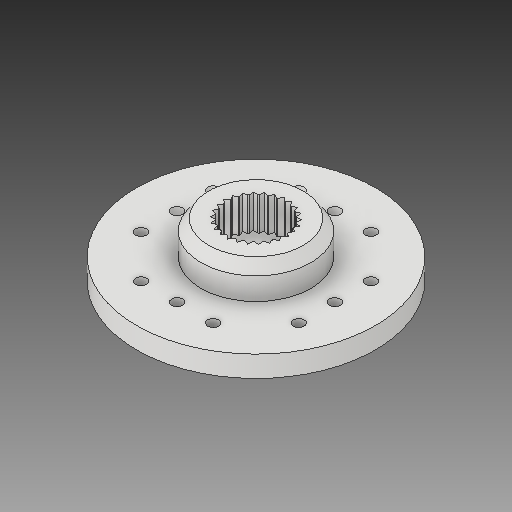
# Autodesk Inventor part: Acople circular
Saved by Autodesk Inventor 2019 (Build 230136000, 136)
## iProperties
Created: 2016-09-27
Part Number: Acople circular
Material: Plástico ABS
Document SubType Name: Modeling
Designer: Julian
Density: 1.06 g/cm^3
Appearance: Suave - Blanco
Mass: 0.859637 g
Surface Area: 11.1715 cm^2
Volume: 0.810978 cm^3
Author: Julian
Autodesk Inventor part; units mm, degrees
ref_plane "YZ Plane" through (0, 0, 0) normal (1, 0, 0) x (0, 1, 0)
ref_plane "XZ Plane" through (0, 0, 0) normal (0, 1, 0) x (-1, 0, 0)
ref_plane "XY Plane" through (0, 0, 0) normal (0, 0, 1) x (1, 0, 0)
sketch "Boceto1" plane through (0, 0, 0) normal (0, 1, 0) x (-1, 0, 0)
  circle A0 centre (0, 0) radius 10.75
  circle A1 centre (7.1, 0) radius 0.5
  circle A2 centre (7.1, -3.25) radius 0.5
  circle A3 centre (7.1, 3.25) radius 0.5
  circle A4 centre (-3.25, 7.1) radius 0.5
  circle A5 centre (0, 7.1) radius 0.5
  circle A6 centre (3.25, 7.1) radius 0.5
  circle A7 centre (-7.1, -3.25) radius 0.5
  circle A8 centre (-7.1, 0) radius 0.5
  circle A9 centre (-7.1, 3.25) radius 0.5
  circle A10 centre (3.25, -7.1) radius 0.5
  circle A11 centre (0, -7.1) radius 0.5
  circle A12 centre (-3.25, -7.1) radius 0.5
  dimension "d0" = 21.5
  dimension "d1" = 1
  dimension "d2" = 6.5
  dimension "d4" = 7.1
  dimension "d7" = 360
  constraints: 13 centre point, 2 equal radius, 1 coincident, 25 other
  measures "d0" diameter of A0
  measures "d1" diameter of A1
  measures "d2" distance of A2.centre A3.centre
  measures "d4" distance of point (0, 0) A1.centre
extrude "Extrusión1" add sketch "Boceto1" along normal blind 1.9
sketch "Boceto2" plane through (0, 1.9, 0) normal (0, 1, 0) x (1, 0, 0)
  circle A0 centre (0, 0) radius 4.95
  dimension "d11" = 9.9
  constraints: 1 centre point, 1 coincident
  measures "d11" diameter of A0
extrude "Extrusión2" add sketch "Boceto2" along normal blind 3
chamfer "Chaflán1" distance 0.7 angle 55 1 edges at (-4.95, 4.9, 0) measured on face at (-4.45, 4.9, 0)
sketch "Boceto6" plane through (0, 0, 0) normal (0, -1, 0) x (1, 0, 0)
  circle A0 centre (0, 0) radius 3.25
  circle A1 centre (0, 0) radius 2.75
  dimension "d24" = 6.5
  dimension "d25" = 0.5
  constraints: 2 centre point, 1 coincident
  measures "d24" diameter of A0
  measures "d25" radial gap between concentric circles of A0 A1
extrude "Extrusión4" add sketch "Boceto6" along normal blind 1
sketch "Boceto7" plane through (0, 0, 0) normal (0, -1, 0) x (1, 0, 0)
  circle A0 centre (0, 0) radius 4.25
  circle A1 centre (0, 0) radius 3.25 projected
  dimension "d28" = 8.5
  constraints: 1 centre point, 1 coincident
  measures "d28" diameter of A0
extrude "Extrusión5" cut sketch "Boceto7" against normal blind 0.4
sketch "Boceto9" plane through (0, 4.9, 0) normal (0, 1, 0) x (1, 0, 0)
  arc A0 (-2.5867, 0.2629) -> (-2.5867, -0.2629) centre (0, 0) ccw
  line L0 (-2.9, 0) -> (-2.5867, -0.2629)
  line L1 (-2.5867, -0.2629) -> (-2.5867, 0.2629)
  line L2 (-2.9, 0) -> (-2.5867, 0.2629)
  dimension "d34" = 5.2
  dimension "d37" = 80
  dimension "d38" = 0.5258
  constraints: 6 end point, 2 point on circle, 1 centre point, 1 coincident
  measures "d34" diameter of A0
  measures "d37" angle of L2 L0
  measures "d38" distance of L0.end L1.end
extrude "Extrusión7" cut sketch "Boceto9" against normal blind 3 contours A0 L0 L2
pattern_circular "Patrón circular1" count 26 over 360 about axis through (0, 4.4001, 0) along (0, 1, 0) of "Extrusión7"
sketch "Boceto10" plane through (0, 4.9, 0) normal (0, 1, 0) x (1, 0, 0)
  arc A0 (-1.6858, -1.9794) -> (-1.253, -2.2781) centre (0, 0) ccw projected
  circle A1 centre (0, 0) radius 2.6
  constraints: 1 centre point, 1 coincident
extrude "Extrusión8" cut sketch "Boceto10" against normal blind 3
sketch "Boceto11" plane through (0, 1.9, 0) normal (0, 1, 0) x (1, 0, 0)
  circle A0 centre (0, 0) radius 1.4
  dimension "d46" = 2.8
  constraints: 1 centre point, 1 coincident
  measures "d46" diameter of A0
extrude "Extrusión9" cut sketch "Boceto11" against normal through all
